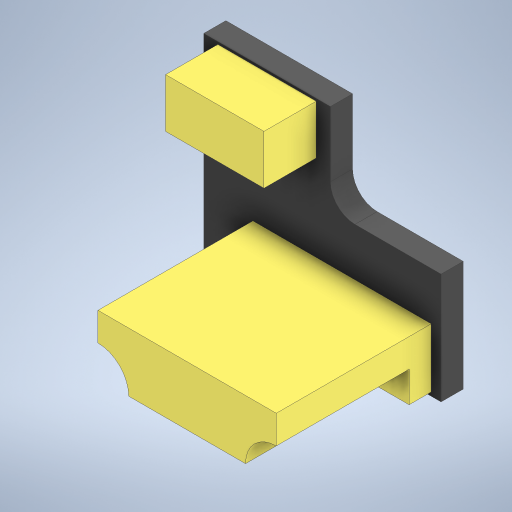
# Autodesk Inventor part: HDMI_Port
Saved by Autodesk Inventor 2023.1 (Build 271208000, 208)
## iProperties
Created: 2022-08-09
Part Number: HDMI_Port
Material: 일반
Document SubType Name: Modeling
Designer: fly01
Density: 1 g/cm^3
Appearance: 기본값
Author: fly01
Autodesk Inventor part; units mm, degrees
ref_plane "YZ Plane" through (0, 0, 0) normal (1, 0, 0) x (0, 1, 0)
ref_plane "XZ Plane" through (0, 0, 0) normal (0, 1, 0) x (-1, 0, 0)
ref_plane "XY Plane" through (0, 0, 0) normal (0, 0, 1) x (1, 0, 0)
sketch "스케치1" plane through (0, 0, 0) normal (0, 0, 1) x (1, 0, 0)
  line L0 (0, 0) -> (19.3, 0)
  line L1 (19.3, 0) -> (19.3, 9)
  line L2 (19.3, 9) -> (10.3, 9)
  line L3 (0, 9) -> (0, 0)
  line L4 (10.3, 9) -> (10.3, 16.3)
  line L5 (10.3, 16.3) -> (0, 16.3)
  line L6 (0, 16.3) -> (0, 9)
  dimension "d0" = 9
  dimension "d1" = 19.3
  dimension "d2" = 16.3
  dimension "d3" = 10.3
  constraints: 14 end point, 3 parallel, 1 horizontal, 1 perpendicular, 1 vertical
  measures "d0" distance of L0.end L1.end
  measures "d1" distance of L0.start L0.end
  measures "d2" distance between parallel lines of L0 L5
  measures "d3" distance of L4.end L5.end
extrude "돌출1" add sketch "스케치1" along normal blind 1.8
fillet "모깎기1" radius 2 1 edges at (10.3, 9, 0.9)
sketch "스케치2" plane through (0, 0, 1.8) normal (0, 0, 1) x (1, 0, 0)
  line L0 (18.5, 0.3) -> (4, 0.3)
  line L1 (4, 0.3) -> (4, 5.1)
  line L2 (4, 5.1) -> (18.5, 5.1)
  line L3 (18.5, 5.1) -> (18.5, 0.3)
  line L4 (19.3, 0) -> (19.3, 9) projected
  line L5 (0, 0) -> (19.3, 0) projected
  line L6 (4, 2.8) -> (4, 2.8)
  line L7 (6.5, 0.3) -> (6.5, 0.3)
  line L8 (6.5, 0.3) -> (16, 0.3)
  line L9 (16, 0.3) -> (16, 0.3)
  line L10 (18.5, 2.8) -> (18.5, 2.8)
  arc A0 (6.5, 0.3) -> (4, 2.8) centre (4, 0.3) ccw
  arc A1 (18.5, 2.8) -> (16, 0.3) centre (18.5, 0.3) ccw
  point P0 (6.5, 2.8)
  point P1 (16, 2.8)
  dimension "d7" = 0.8
  dimension "d8" = 14.5
  dimension "d9" = 4.8
  dimension "d10" = 0.3
  dimension "d11" = 2.3
  dimension "d12" = 2.5
  dimension "d13" = 2.5
  dimension "d14" = 2.5
  dimension "d15" = 2.5
  constraints: 18 end point, 8 point on line, 5 perpendicular, 4 point on circle, 4 tangent, 2 centre point, 2 parallel, 1 equal radius, 1 horizontal
  measures "d7" distance between parallel lines of L4 L3
  measures "d8" distance of L0.start L0.end
  measures "d9" distance of L2.end L0.start
  measures "d10" distance between parallel lines of L5 L0
  measures "d11" distance between parallel lines of L2 L10
  measures "d12" distance of L8.end point (16, 2.8)
  measures "d13" distance of L6.start point (6.5, 2.8)
  measures "d14" distance of point (16, 2.8) L10.end
  measures "d15" radius of A0
extrude "돌출2" add sketch "스케치2" along normal blind 12.6 contours L0 A0 L1 L2 L3 A1
extrude "돌출3" add sketch "스케치2" along normal blind 1.8 contours L0 A1 L3 | L0 L1 A0
sketch "스케치3" plane through (0, 0, 1.8) normal (0, 0, 1) x (1, 0, 0)
  line L0 (1.15, 16.1) -> (9.15, 16.1)
  line L1 (9.15, 16.1) -> (9.15, 12.1)
  line L2 (9.15, 12.1) -> (1.15, 12.1)
  line L3 (1.15, 12.1) -> (1.15, 16.1)
  line L4 (10.3, 16.3) -> (0, 16.3) projected
  point P0 (0, 0)
  point P1 (5.15, 16.1)
  point P2 (5.15, 16.3)
  dimension "d20" = 8
  dimension "d21" = 4
  dimension "d22" = 0.2
  constraints: 8 end point, 2 midpoint, 2 parallel, 1 horizontal, 1 perpendicular, 1 vertical alignment
  measures "d20" distance of L0.start L0.end
  measures "d21" distance of L0.end L1.end
  measures "d22" distance between parallel lines of L4 L0
extrude "돌출4" add sketch "스케치3" along normal blind 4.25
